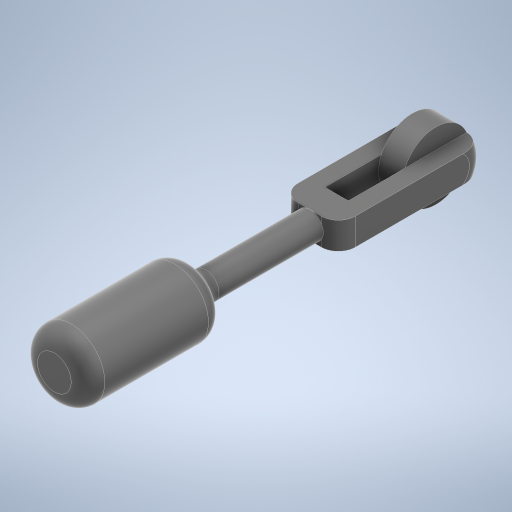
# Autodesk Inventor part: joint_v2
Saved by Autodesk Inventor 2023 (Build 270158000, 158)
## iProperties
Created: 2022-11-07
Part Number: joint_v2
Material: 일반
Document SubType Name: Modeling
Designer: willy
Density: 1 g/cm^3
Appearance: 매끄러움 - 검은색
Author: willy
Autodesk Inventor part; units mm, degrees
ref_plane "YZ Plane" through (0, 0, 0) normal (1, 0, 0) x (0, 1, 0)
ref_plane "XZ Plane" through (0, 0, 0) normal (0, 1, 0) x (-1, 0, 0)
sketch "스케치1" plane through (0, 0, 0) normal (0, 0, 1) x (1, 0, 0)
  circle A0 centre (0, 0) radius 10
  dimension "d0" = 20
  constraints: 1 centre point, 1 coincident
  measures "d0" diameter of A0
extrude "돌출1" add sketch "스케치1" against normal blind 40
sketch "스케치2" plane through (0, 0, -40) normal (0, 0, -1) x (-1, 0, 0)
  circle A0 centre (0, 0) radius 4
  dimension "d3" = 8
  constraints: 1 centre point, 1 coincident
  measures "d3" diameter of A0
extrude "돌출2" add sketch "스케치2" along normal blind 40
sketch "스케치3" plane through (0, 0, 0) normal (0, 1, 0) x (-1, 0, 0)
  line L0 (-4, -80) -> (4, -80) projected
  line L1 (0, -80) -> (7.5, -80)
  line L2 (7.5, -80) -> (7.5, -120)
  line L3 (0, -80) -> (-7.5, -80)
  line L4 (-7.5, -80) -> (-7.5, -120)
  point P0 (0, 0)
  dimension "d6" = 7.5
  dimension "d7" = 7.5
  dimension "d8" = 40
  dimension "d9" = 40
  constraints: 8 end point, 2 perpendicular, 1 horizontal, 1 midpoint, 1 point on line
  measures "d6" distance of L1.start L1.end
  measures "d7" distance of L1.start L3.end
  measures "d8" distance of L1.end L2.end
  measures "d9" distance of L3.end L4.end
ref_plane "작업 평면1" through (7.5, 0, -120) normal (0, 0, -1) x (-1, 0, 0)
sketch "스케치4" plane through (7.5, 0, -120) normal (0, 0, -1) x (-1, 0, 0)
  line L0 (-4, -4) -> (4, -4)
  line L1 (4, -4) -> (4, 4)
  line L2 (4, 4) -> (-4, 4)
  line L3 (-4, 4) -> (-4, -4)
  line L4 (-4, -4) -> (4, 4) construction
  line L5 (4, -4) -> (-4, 4) construction
  point P0 (7.5, 0)
  point P1 (0, 0)
  dimension "d10" = 8
  dimension "d11" = 8
  constraints: 12 end point, 2 midpoint, 2 parallel, 1 horizontal, 1 perpendicular
  measures "d10" distance of L2.end L1.end
  measures "d11" distance of L1.end L0.end
sweep "스윕1" add profiles "스케치4" path "스케치3" path curves L4 L3 L1 L2
sketch "스케치6" plane through (3.5, -4, -120) normal (-1, 0, 0) x (0, 0, 1)
  circle A0 centre (10, 4) radius 10
  line L0 (0, 0) -> (0, 8) projected
  line L1 (0, 0) -> (44, 0) projected
  line L2 (0.8348, 0) -> (0, 0)
  line L3 (0, 8) -> (0, 0) projected
  line L4 (0, 4) -> (0, 0)
  line L5 (0, 8) -> (44, 8) projected
  line L6 (0, 4) -> (0, 8)
  line L7 (0, 8) -> (0.8348, 8)
  point P0 (120, 4)
  point P1 (5, 0)
  point P2 (39, 0)
  point P3 (39, 8)
  point P4 (0.8348, 8)
  point P5 (0, 4)
  dimension "d18" = 20
  dimension "d19" = 4
  constraints: 8 end point, 2 point on circle, 1 centre point, 1 collinear, 1 midpoint, 1 perpendicular, 1 point on line, 1 tangent, 1 vertical
  measures "d18" diameter of A0
  measures "d19" distance from line of L1 A0.centre
fillet "모깎기2" radius 5 1 edges at (4, 0, -40)
fillet "모깎기4" radius 5 2 edges at (-10, 0, 0) (-10, 0, -40)
extrude "돌출4" add sketch "스케치6" along normal blind 7 contours L5 A0 L1 | A0 L5 | L1 A0
extrude "돌출3" cut sketch "스케치6" along normal through all both and the other way through all contours A0 L0 L5 | A0 L1 L0
sketch "스케치9" plane through (-11.5, 4, -76) normal (0, 1, 0) x (1, 0, 0)
  line L0 (11.5, 0) -> (0, 0) projected
  line L1 (3, 0) -> (3, 44)
  line L2 (23, 44) -> (0, 44) projected
  line L3 (0, 0) -> (0, 43.1652) projected
  line L4 (23, 0) -> (11.5, 0) projected
  line L5 (20, 0) -> (20, 44)
  line L6 (23, 43.1652) -> (23, 0) projected
  line L7 (3, 0) -> (0, 0)
  line L8 (0, 44) -> (0, 0)
  line L9 (3, 44) -> (0, 44)
  line L10 (20, 0) -> (23, 0)
  line L11 (23, 0) -> (23, 44)
  line L12 (23, 43.1652) -> (23, 44) projected
  line L13 (23, 44) -> (20, 44)
  point P0 (11.5, -76)
  dimension "d30" = 3
  dimension "d31" = 3
  constraints: 16 end point, 5 collinear, 4 point on line, 2 perpendicular, 1 vertical
  measures "d30" distance between parallel lines of L3 L1
  measures "d31" distance between parallel lines of L6 L5
extrude "돌출6" cut sketch "스케치9" against normal through all contours L0 L3 L8 L2 L1 | L5 L2 L11 L6 L4
fillet "모깎기6" radius 5 6 edges at (8.5, 0, -76) (-8.5, 0, -76) (8.5, -2.0431, -119.7891) (8.5, 2.0431, -119.7891) (-8.5, -2.0431, -119.7891) (-8.5, 2.0431, -119.7891)
